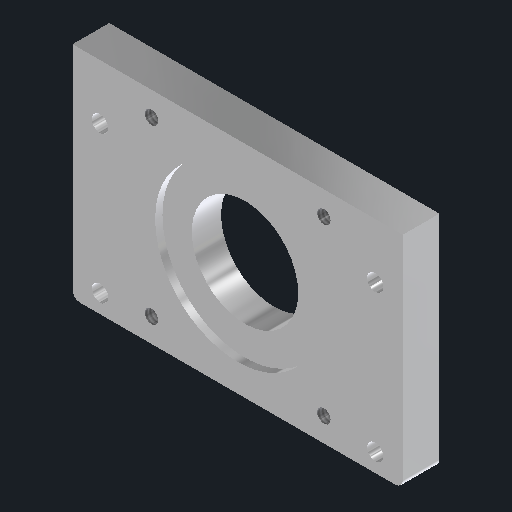
# Autodesk Inventor part: MonturaMotor
Saved by Autodesk Inventor 2022 (Build 260153000, 153)
## iProperties
Created: 2021-09-22
Part Number: MonturaMotor
Material: Aluminum 6061
Document SubType Name: Modeling
Designer: Andres
Density: 2.7 g/cm^3
Appearance: Aluminum - Flat
Author: Andres
Autodesk Inventor part; units mm, degrees
ref_plane "YZ Plane" through (0, 0, 0) normal (1, 0, 0) x (0, 1, 0)
ref_plane "XZ Plane" through (0, 0, 0) normal (0, 1, 0) x (-1, 0, 0)
ref_plane "XY Plane" through (0, 0, 0) normal (0, 0, 1) x (1, 0, 0)
sketch "Sketch1" plane through (0, 0, 0) normal (0, 0, 1) x (1, 0, 0)
  line L0 (115, 10) -> (137, 10) projected
  line L1 (137, -48) -> (3, -48) projected
  line L2 (3, 10) -> (25, 10) projected
  circle A0 centre (70, -10) radius 12.5 projected
  circle A1 centre (70, -10) radius 14.5
  arc A2 (113, -40) -> (115, -38) centre (113, -38) ccw projected
  line L3 (113, -40) -> (27, -40) projected
  arc A3 (25, -38) -> (27, -40) centre (27, -38) ccw projected
  line L4 (115, 10) -> (115, -38) projected
  line L5 (25, -38) -> (25, 10) projected
  line L6 (25, 10) -> (25, 20)
  line L7 (25, 20) -> (115, 20)
  line L8 (115, 20) -> (115, 10)
  line L9 (3, -48) -> (3, 10) projected
  line L10 (137, 10) -> (137, -48) projected
  dimension "d1" = 2
  dimension "d6" = 30
  dimension "d7" = 30
  constraints: 6 end point, 2 perpendicular, 1 centre point, 1 vertical
  measures "d1" radial gap between concentric circles of A0 A1
  measures "d6" distance from line of A0.centre L7
  measures "d7" distance from line of L3 A0.centre
extrude "Extrusion1" add sketch "Sketch1" along normal mid plane 8 contours L4 A2 L3 A3 L5 L6 L7 L8
sketch "Sketch6" plane through (0, 0, 4) normal (0, 0, 1) x (1, 0, 0)
  circle A0 centre (70, -10) radius 14.5 projected
  circle A1 centre (70, -10) radius 22.5
  line L0 (115, 20) -> (25, 20) projected
  line L1 (25, 20) -> (25, -38) projected
  arc A2 (25, -38) -> (27, -40) centre (27, -38) ccw projected
  line L2 (27, -40) -> (113, -40) projected
  arc A3 (113, -40) -> (115, -38) centre (113, -38) ccw projected
  line L3 (115, -38) -> (115, 20) projected
  circle A4 centre (70, -10) radius 14.5 projected
  point P0 (0, 0)
  dimension "d25" = 45
  constraints: 1 centre point, 1 coincident
  measures "d25" diameter of A1
extrude "Extrusion2" add sketch "Sketch6" along normal blind 2 contours L3 A3 L2 A2 L1 L0
sketch "Sketch5" plane through (0, 0, 6) normal (0, 0, 1) x (1, 0, 0)
  circle A0 centre (46.5, 13.5) radius 2.5 projected
  circle A1 centre (46.5, -33.5) radius 2.5 projected
  circle A2 centre (93.5, 13.5) radius 2.5 projected
  circle A3 centre (93.5, -33.5) radius 2.5 projected
  point P0 (0, 0)
hole "Hole2" at (46.5, 13.5, 6) at (46.5, -33.5, 6) at (93.5, -33.5, 6) at (93.5, 13.5, 6) direction (0, 0, -1) diameter 3.683 depth 6 tip angle 118 thread size "10-24 UNC" class "2B" standard "ANSI Unified Screw Threads"
sketch "Sketch7" plane through (0, 0, 6) normal (0, 0, 1) x (1, 0, 0)
  circle A0 centre (70, -10) radius 14.5 projected
  line L0 (32.5, -35) -> (107.5, -35) construction
  line L1 (107.5, -35) -> (107.5, 5) construction
  line L2 (107.5, 5) -> (32.5, 5) construction
  line L3 (32.5, 5) -> (32.5, -35) construction
  line L4 (32.5, -35) -> (107.5, 5) construction
  line L5 (107.5, -35) -> (32.5, 5) construction
  point P0 (0, 0)
  point P1 (70, -15)
  point P2 (70, -15)
  dimension "d28" = 75
  dimension "d29" = 40
  dimension "d30" = 5
  constraints: 12 end point, 3 midpoint, 2 parallel, 1 horizontal, 1 perpendicular, 1 vertical alignment
  measures "d28" distance of L1.end L2.end
  measures "d29" distance of L2.end L0.start
  measures "d30" distance of A0.centre point (70, -15)
hole "Hole3" at (32.5, 5, 6) at (32.5, -35, 6) at (107.5, -35, 6) at (107.5, 5, 6) direction (0, 0, -1) diameter 4.5 end through all clearance for "Socket Head Cap Screw ISO 4762" size "M4" standard "ISO"
equation "\"d6\" = d7"
body "Solid1"
